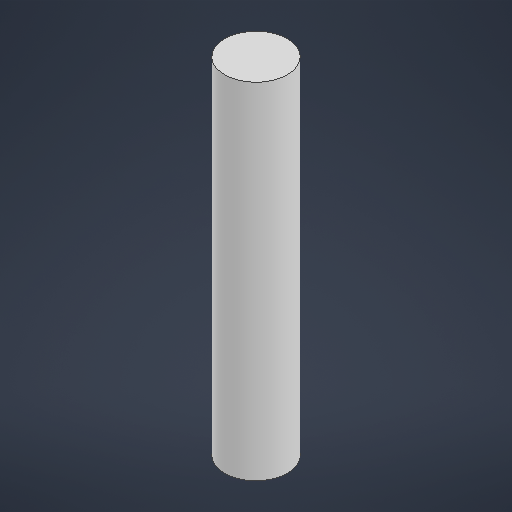
# Autodesk Inventor part: Part1
Saved by Autodesk Inventor 2026.1 (Build 301233000, 233)
## iProperties
Created: 2026-09-23
Part Number: Part1
Material: Generic
Document SubType Name: Modeling
Designer: share
Density: 1 g/cm^3
Appearance: Default
Author: share
Autodesk Inventor part; units mm, degrees
ref_plane "YZ Plane" through (0, 0, 0) normal (1, 0, 0) x (0, 1, 0)
ref_plane "XZ Plane" through (0, 0, 0) normal (0, 1, 0) x (-1, 0, 0)
ref_plane "XY Plane" through (0, 0, 0) normal (0, 0, 1) x (1, 0, 0)
sketch "Sketch1" plane through (0, 0, 0) normal (0, 1, 0) x (-1, 0, 0)
  circle A0 centre (0, 0) radius 6.35
  dimension "d0" = 12.7
  constraints: 1 centre point, 1 coincident
  measures "d0" diameter of A0
extrude "Extrusion1" add sketch "Sketch1" along normal mid plane 70
body "Solid1"
